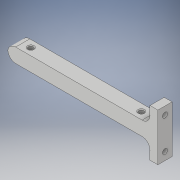
# Autodesk Inventor part: PCB_STAND
Saved by Autodesk Inventor 2019 (Build 230136000, 136)
## iProperties
Created: 2021-11-23
Part Number: PCB_STAND
Material: Generic
Document SubType Name: Modeling
Designer: Pokick
Density: 1 g/cm^3
Appearance: Default
Author: Pokick
Autodesk Inventor part; units mm, degrees
ref_plane "YZ Plane" through (0, 0, 0) normal (1, 0, 0) x (0, 1, 0)
ref_plane "XZ Plane" through (0, 0, 0) normal (0, 1, 0) x (-1, 0, 0)
ref_plane "XY Plane" through (0, 0, 0) normal (0, 0, 1) x (1, 0, 0)
sketch "Sketch1" plane through (0, 0, 0) normal (0, 1, 0) x (-1, 0, 0)
  line L0 (-35, 45) -> (35, 45) construction
  line L1 (35, 45) -> (35, -45) construction
  line L2 (35, -45) -> (-35, -45) construction
  line L3 (-35, -45) -> (-35, 45) construction
  line L4 (-35, 45) -> (35, -45) construction
  line L5 (35, 45) -> (-35, -45) construction
  circle A0 centre (35, 45) radius 1.6
  circle A1 centre (35, -45) radius 1.6 construction
  circle A2 centre (-35, -45) radius 1.6 construction
  circle A3 centre (-35, 45) radius 1.6
  line L6 (-45, 49.5) -> (45, 49.5)
  line L7 (45, 49.5) -> (45, 40.5)
  line L8 (45, 40.5) -> (-45, 40.5)
  line L9 (-45, 40.5) -> (-45, 49.5)
  line L10 (-45, 49.5) -> (45, 40.5) construction
  line L11 (45, 49.5) -> (-45, 40.5) construction
  point P0 (0, 0)
  point P1 (0, 45)
  dimension "d0" = 70
  dimension "d1" = 90
  dimension "d2" = 3.2
  dimension "d3" = 3.2
  dimension "d4" = 3.2
  dimension "d5" = 3.2
  dimension "d6" = 90
  dimension "d7" = 9
  constraints: 24 end point, 5 midpoint, 4 centre point, 4 coincident, 4 parallel, 2 horizontal, 2 perpendicular
  measures "d0" distance of L1.end L2.end
  measures "d1" distance of L0.end L1.end
  measures "d2" diameter of A0
  measures "d3" diameter of A3
  measures "d4" diameter of A1
  measures "d5" diameter of A2
  measures "d6" distance of L7.end L8.end
  measures "d7" distance of L6.end L7.end
extrude "Extrusion1" add sketch "Sketch1" along normal mid plane 9
sketch "Sketch2" plane through (45, -4.5, 40.5) normal (1, 0, 0) x (0, 0, -1)
  line L0 (0, 0) -> (-9, 0) construction
  line L1 (0, 0) -> (-9, 0) construction
  line L2 (-9, 0) -> (-9, 9) construction
  line L3 (-9, 9) -> (0, 9) construction
  line L4 (0, 9) -> (0, 0) construction
  line L5 (-9, 0) -> (-9, 9) construction
  line L6 (-9, 0) -> (0, 9) construction
  line L7 (-9, 9) -> (0, 9) construction
  line L8 (-9, 9) -> (0, 0) construction
  line L9 (-9, -10.5) -> (0, -10.5)
  line L10 (0, -10.5) -> (0, 19.5)
  line L11 (0, 19.5) -> (-9, 19.5)
  line L12 (-9, 19.5) -> (-9, -10.5)
  line L13 (-9, -10.5) -> (0, 19.5) construction
  line L14 (0, -10.5) -> (-9, 19.5) construction
  line L15 (-4.5, 4.5) -> (-4.5, 14.5) construction
  line L16 (-4.5, 4.5) -> (-4.5, -5.5) construction
  circle A0 centre (-4.5, 14.5) radius 1.6
  circle A1 centre (-4.5, -5.5) radius 1.6
  point P0 (40.5, 4.5)
  dimension "d10" = 9
  dimension "d11" = 30
  dimension "d12" = 10
  dimension "d13" = 10
  dimension "d14" = 3.2
  dimension "d15" = 3.2
  constraints: 28 end point, 4 parallel, 3 midpoint, 3 perpendicular, 2 centre point, 2 coincident, 2 horizontal, 2 vertical
  measures "d10" distance of L11.end L10.end
  measures "d11" distance of L10.end L9.end
  measures "d12" distance of L15.start L15.end
  measures "d13" distance of L15.start L16.end
  measures "d14" diameter of A0
  measures "d15" diameter of A1
extrude "Extrusion2" add sketch "Sketch2" along normal blind 5
fillet "Fillet1" radius 5 2 edges at (45, -4.5, 45) (45, 4.5, 45)
fillet "Fillet2" radius 5 2 edges at (-45, -4.5, 45) (-45, 4.5, 45)
fillet "Fillet3" radius 1 6 edges at (44.8775, 8.4, 45) (45, 9.7468, 43.4202) (45, 11.5798, 45.2532) (44.8775, -8.4, 45) (45, -11.5798, 45.2532) (45, -9.7468, 43.4202)
fillet "Fillet4" radius 0.5 4 edges at (36.6, -4.5, 45) (-33.4, -4.5, 45) (-33.4, 4.5, 45) (36.6, 4.5, 45)
equation "\"d3\" = d2"
equation "\"d4\" = d2"
equation "\"d5\" = d2"
body "Solid1"
